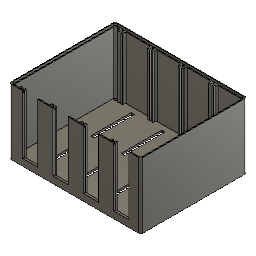
clusterbox-rock64-3d-v18 (Autodesk Fusion 360 design; units mm, degrees)
Autodesk Fusion 360 part; units mm, degrees
sketch "Sketch1" plane through (0, 0, 0) normal (0, 1, 0) x (1, 0, 0)
  line L0 (-65, -52.5) -> (65, -52.5)
  line L1 (65, -52.5) -> (65, 52.5)
  line L2 (65, 52.5) -> (-65, 52.5)
  line L3 (-65, 52.5) -> (-65, -52.5)
  line L4 (-65, -52.5) -> (65, 52.5) construction
  line L5 (65, -52.5) -> (-65, 52.5) construction
  dimension "d1" = 105
  dimension "d2" = 130
extrude "Extrude1" add sketch "Sketch1" along normal blind 65
sketch "Sketch2" plane through (0, 65, 0) normal (0, 1, 0) x (-1, 0, 0)
  line L0 (65, -52.5) -> (65, 52.5)
  line L1 (65, 52.5) -> (-65, 52.5)
  line L2 (-65, 52.5) -> (-65, -52.5)
  line L3 (-65, -52.5) -> (65, -52.5)
  line L4 (63, 50.5) -> (-63, 50.5)
  line L5 (-63, 50.5) -> (-63, -50.5)
  line L6 (-63, -50.5) -> (63, -50.5)
  line L7 (63, -50.5) -> (63, 50.5)
  line L8 (63, 50.5) -> (-63, -50.5) construction
  line L9 (-63, 50.5) -> (63, -50.5) construction
  dimension "d5" = 2
  dimension "d6" = 2
  measures "d5" distance of L0 L7
  measures "d6" distance of L1 L4
extrude "Extrude2" cut sketch "Sketch2" against normal blind 63 contours L4 L5 L6 L7
sketch "Sketch3" plane through (0, 2, 0) normal (0, 1, 0) x (-1, 0, 0)
  line L0 (63, -50.5) -> (63, 50.5)
  line L1 (63, 50.5) -> (-63, 50.5)
  line L2 (-63, 50.5) -> (-63, -50.5)
  line L3 (-63, -50.5) -> (63, -50.5)
  line L4 (58, -50.5) -> (53, -50.5)
  line L5 (53, -50.5) -> (53, -47.5)
  line L6 (53, -47.5) -> (58, -47.5)
  line L7 (58, -47.5) -> (58, -50.5)
  line L8 (63, 50.5) -> (63, -50.5)
  line L9 (65, -52.5) -> (65, 52.5) construction
  line L10 (-65, 52.5) -> (-65, -52.5) construction
  line L11 (65, 0) -> (-65, 0) construction
  line L12 (58, 50.5) -> (53, 50.5)
  line L13 (58, 47.5) -> (58, 50.5)
  line L14 (53, 47.5) -> (58, 47.5)
  line L15 (53, 50.5) -> (53, 47.5)
  dimension "d9" = 5
  dimension "d10" = 3
  dimension "d11" = 5
  measures "d11" distance of L7 L8
extrude "Extrude3" add sketch "Sketch3" along normal blind 63 contours L3 L4 L5 L6 L7 | L1 L12 L13 L14 L15
sketch "Sketch4" plane through (0, 2, 0) normal (0, 1, 0) x (-1, 0, 0)
  line L0 (58, 50.5) -> (58, 47.5)
  line L1 (58, 47.5) -> (53, 47.5)
  line L2 (53, 47.5) -> (53, 50.5)
  line L3 (53, 50.5) -> (-63, 50.5)
  line L4 (-63, 50.5) -> (-63, -50.5)
  line L5 (-63, -50.5) -> (53, -50.5)
  line L6 (53, -50.5) -> (53, -47.5)
  line L7 (53, -47.5) -> (58, -47.5)
  line L8 (58, -47.5) -> (58, -50.5)
  line L9 (58, -50.5) -> (63, -50.5)
  line L10 (63, -50.5) -> (63, 50.5)
  line L11 (63, 50.5) -> (58, 50.5)
  line L12 (56.375, -50.5) -> (54.625, -50.5)
  line L13 (54.625, -50.5) -> (54.625, 50.5)
  line L14 (54.625, 50.5) -> (56.375, 50.5)
  line L15 (56.375, 50.5) -> (56.375, -50.5)
  line L16 (0, 0) -> (54.625, 0) construction
  line L17 (58, -50.5) -> (58, -47.5) construction
  line L18 (55.5, -47.5) -> (55.5, -51.2811) construction
  dimension "d14" = 1.75
  dimension "d16" = 101
  measures "d14" distance of L13 L15
extrude "Extrude4" cut sketch "Sketch4" along normal blind 63 contours L1 L7 L13 L15 | L1 L13 L14 L15 | L7 L12 L13 L15
fillet "Fillet1" radius 1.5 4 edges at (-58, 33.5, 50.5) (-53, 33.5, 50.5) (-53, 33.5, -50.5) (-58, 33.5, -50.5)
pattern_linear "R-Pattern1" count 4 spacing 30 along (1, 0, 0) of "Extrude3", "Extrude4", "Fillet1"
fillet "Fillet2" radius 2 4 edges at (65, 32.5, -52.5) (65, 32.5, 52.5) (-65, 32.5, 52.5) (-65, 32.5, -52.5)
fillet "Fillet2" radius 2 4 edges at (63, 33.5, -50.5) (-63, 33.5, -50.5) (-63, 33.5, 50.5) (63, 33.5, 50.5)
sketch "Sketch5" plane through (0, 0, 0) normal (0, -1, 0) x (1, 0, 0)
  arc A0 (-65, -50.5) -> (-63, -52.5) centre (-63, -50.5) ccw
  line L0 (-63, -52.5) -> (63, -52.5)
  arc A1 (63, -52.5) -> (65, -50.5) centre (63, -50.5) ccw
  line L1 (65, -50.5) -> (65, 50.5)
  arc A2 (65, 50.5) -> (63, 52.5) centre (63, 50.5) ccw
  line L2 (63, 52.5) -> (-63, 52.5)
  arc A3 (-63, 52.5) -> (-65, 50.5) centre (-63, 50.5) ccw
  line L3 (-65, 50.5) -> (-65, -50.5)
  line L4 (-65, 48.5) -> (65, 48.5) construction
  line L5 (-65, 0) -> (65, 0) construction
  circle A4 centre (-61, 48.5) radius 1.1
  circle A5 centre (-61, -48.5) radius 1.1
  line L6 (0, 52.5) -> (0, 0) construction
  circle A6 centre (61, 48.5) radius 1.1
  circle A7 centre (61, -48.5) radius 1.1
  dimension "d29" = 2.2
  dimension "d36" = 4
  dimension "d37" = 4
  measures "d29" diameter of A4
extrude "Extrude5" cut sketch "Sketch5" against normal blind 2 contours A4 | A5 | A6 | A7
sketch "Sketch7" plane through (0, 2, 0) normal (0, 1, 0) x (-1, 0, 0)
  circle A0 centre (61, 48.5) radius 1.1
  circle A1 centre (61, -48.5) radius 1.1
  circle A2 centre (-61, 48.5) radius 1.1
  circle A3 centre (-61, -48.5) radius 1.1
  arc A4 (-61, 50.5) -> (-63, 48.5) centre (-61, 48.5) ccw
  line L0 (-63, 48.5) -> (-63, -48.5)
  arc A5 (-63, -48.5) -> (-61, -50.5) centre (-61, -48.5) ccw
  line L1 (-61, -50.5) -> (-38.5, -50.5)
  arc A6 (-38.5, -50.5) -> (-37, -49) centre (-38.5, -49) ccw
  line L2 (-37, -49) -> (-37, -47.5)
  line L3 (-37, -47.5) -> (-35.375, -47.5)
  line L4 (-35.375, -47.5) -> (-35.375, -50.5)
  line L5 (-35.375, -50.5) -> (-33.625, -50.5)
  line L6 (-33.625, -50.5) -> (-33.625, -47.5)
  line L7 (-33.625, -47.5) -> (-32, -47.5)
  line L8 (-32, -47.5) -> (-32, -49)
  arc A7 (-32, -49) -> (-30.5, -50.5) centre (-30.5, -49) ccw
  line L9 (-30.5, -50.5) -> (-8.5, -50.5)
  arc A8 (-8.5, -50.5) -> (-7, -49) centre (-8.5, -49) ccw
  line L10 (-7, -49) -> (-7, -47.5)
  line L11 (-7, -47.5) -> (-5.375, -47.5)
  line L12 (-5.375, -47.5) -> (-5.375, -50.5)
  line L13 (-5.375, -50.5) -> (-3.625, -50.5)
  line L14 (-3.625, -50.5) -> (-3.625, -47.5)
  line L15 (-3.625, -47.5) -> (-2, -47.5)
  line L16 (-2, -47.5) -> (-2, -49)
  arc A9 (-2, -49) -> (-0.5, -50.5) centre (-0.5, -49) ccw
  line L17 (-0.5, -50.5) -> (21.5, -50.5)
  arc A10 (21.5, -50.5) -> (23, -49) centre (21.5, -49) ccw
  line L18 (23, -49) -> (23, -47.5)
  line L19 (23, -47.5) -> (24.625, -47.5)
  line L20 (24.625, -47.5) -> (24.625, -50.5)
  line L21 (24.625, -50.5) -> (26.375, -50.5)
  line L22 (26.375, -50.5) -> (26.375, -47.5)
  line L23 (26.375, -47.5) -> (28, -47.5)
  line L24 (28, -47.5) -> (28, -49)
  arc A11 (28, -49) -> (29.5, -50.5) centre (29.5, -49) ccw
  line L25 (54.625, -47.5) -> (54.625, -50.5)
  line L26 (54.625, -50.5) -> (56.375, -50.5)
  line L27 (56.375, -50.5) -> (56.375, -47.5)
  line L28 (56.375, -47.5) -> (58, -47.5)
  line L29 (58, -47.5) -> (58, -49)
  arc A12 (58, -49) -> (59.5, -50.5) centre (59.5, -49) ccw
  line L30 (59.5, -50.5) -> (61, -50.5)
  arc A13 (61, -50.5) -> (63, -48.5) centre (61, -48.5) ccw
  line L31 (63, -48.5) -> (63, 48.5)
  arc A14 (63, 48.5) -> (61, 50.5) centre (61, 48.5) ccw
  line L32 (61, 50.5) -> (59.5, 50.5)
  arc A15 (59.5, 50.5) -> (58, 49) centre (59.5, 49) ccw
  line L33 (58, 49) -> (58, 47.5)
  line L34 (58, 47.5) -> (56.375, 47.5)
  line L35 (56.375, 47.5) -> (56.375, 50.5)
  line L36 (56.375, 50.5) -> (54.625, 50.5)
  line L37 (54.625, 50.5) -> (54.625, 47.5)
  arc A16 (29.5, 50.5) -> (28, 49) centre (29.5, 49) ccw
  line L38 (28, 49) -> (28, 47.5)
  line L39 (28, 47.5) -> (26.375, 47.5)
  line L40 (26.375, 47.5) -> (26.375, 50.5)
  line L41 (26.375, 50.5) -> (24.625, 50.5)
  line L42 (24.625, 50.5) -> (24.625, 47.5)
  line L43 (24.625, 47.5) -> (23, 47.5)
  line L44 (23, 47.5) -> (23, 49)
  arc A17 (23, 49) -> (21.5, 50.5) centre (21.5, 49) ccw
  line L45 (21.5, 50.5) -> (-0.5, 50.5)
  arc A18 (-0.5, 50.5) -> (-2, 49) centre (-0.5, 49) ccw
  line L46 (-2, 49) -> (-2, 47.5)
  line L47 (-2, 47.5) -> (-3.625, 47.5)
  line L48 (-3.625, 47.5) -> (-3.625, 50.5)
  line L49 (-3.625, 50.5) -> (-5.375, 50.5)
  line L50 (-5.375, 50.5) -> (-5.375, 47.5)
  line L51 (-5.375, 47.5) -> (-7, 47.5)
  line L52 (-7, 47.5) -> (-7, 49)
  arc A19 (-7, 49) -> (-8.5, 50.5) centre (-8.5, 49) ccw
  line L53 (-8.5, 50.5) -> (-30.5, 50.5)
  arc A20 (-30.5, 50.5) -> (-32, 49) centre (-30.5, 49) ccw
  line L54 (-32, 49) -> (-32, 47.5)
  line L55 (-32, 47.5) -> (-33.625, 47.5)
  line L56 (-33.625, 47.5) -> (-33.625, 50.5)
  line L57 (-33.625, 50.5) -> (-35.375, 50.5)
  line L58 (-35.375, 50.5) -> (-35.375, 47.5)
  line L59 (-35.375, 47.5) -> (-37, 47.5)
  line L60 (-37, 47.5) -> (-37, 49)
  arc A21 (-37, 49) -> (-38.5, 50.5) centre (-38.5, 49) ccw
  line L61 (-38.5, 50.5) -> (-61, 50.5)
  line L62 (63, 0) -> (-63, 0) construction
  line L63 (51.5, -50.5) -> (29.5, -50.5) construction
  line L64 (40.5, -50.5) -> (40.5, 0) construction
  line L65 (42.1, -5.25) -> (38.9, -5.25)
  line L66 (38.9, -5.25) -> (38.9, -45.25)
  line L67 (38.9, -45.25) -> (42.1, -45.25)
  line L68 (42.1, -45.25) -> (42.1, -5.25)
  line L69 (42.1, -5.25) -> (38.9, -45.25) construction
  line L70 (38.9, -5.25) -> (42.1, -45.25) construction
  line L71 (42.1, 45.25) -> (42.1, 5.25)
  line L72 (38.9, 45.25) -> (42.1, 45.25)
  line L73 (38.9, 5.25) -> (38.9, 45.25)
  line L74 (42.1, 5.25) -> (38.9, 5.25)
  dimension "d51" = 3.2
  dimension "d52" = 40
  measures "d52" distance of origin
extrude "Extrude6" cut sketch "Sketch7" against normal through all contours L65 L66 L67 L68 | L71 L72 L73 L74
pattern_linear "R-Pattern2" count 4 spacing 30 along (1, 0, 0) of "Extrude6"
sketch "Sketch6" plane through (0, 65, 0) normal (0, 1, 0) x (-1, 0, 0)
  arc A0 (63, -52.5) -> (65, -50.5) centre (63, -50.5) ccw
  line L0 (65, -50.5) -> (65, 50.5)
  arc A1 (65, 50.5) -> (63, 52.5) centre (63, 50.5) ccw
  line L1 (63, 52.5) -> (-63, 52.5)
  arc A2 (-63, 52.5) -> (-65, 50.5) centre (-63, 50.5) ccw
  line L2 (-65, 50.5) -> (-65, -50.5)
  arc A3 (-65, -50.5) -> (-63, -52.5) centre (-63, -50.5) ccw
  line L3 (-63, -52.5) -> (63, -52.5)
  line L4 (-33.625, -47.5) -> (-33.625, -50.5)
  line L5 (-33.625, -50.5) -> (-35.375, -50.5)
  line L6 (-35.375, -50.5) -> (-35.375, -47.5)
  line L7 (-35.375, -47.5) -> (-37, -47.5)
  line L8 (-37, -47.5) -> (-37, -49)
  arc A4 (-38.5, -50.5) -> (-37, -49) centre (-38.5, -49) ccw
  line L9 (-38.5, -50.5) -> (-61, -50.5)
  arc A5 (-63, -48.5) -> (-61, -50.5) centre (-61, -48.5) ccw
  line L10 (-63, -48.5) -> (-63, 48.5)
  arc A6 (-61, 50.5) -> (-63, 48.5) centre (-61, 48.5) ccw
  line L11 (-61, 50.5) -> (-38.5, 50.5)
  arc A7 (-37, 49) -> (-38.5, 50.5) centre (-38.5, 49) ccw
  line L12 (-37, 49) -> (-37, 47.5)
  line L13 (-37, 47.5) -> (-35.375, 47.5)
  line L14 (-35.375, 47.5) -> (-35.375, 50.5)
  line L15 (-35.375, 50.5) -> (-33.625, 50.5)
  line L16 (-33.625, 50.5) -> (-33.625, 47.5)
  line L17 (-33.625, 47.5) -> (-32, 47.5)
  line L18 (-32, 47.5) -> (-32, 49)
  arc A8 (-30.5, 50.5) -> (-32, 49) centre (-30.5, 49) ccw
  line L19 (-30.5, 50.5) -> (-8.5, 50.5)
  arc A9 (-7, 49) -> (-8.5, 50.5) centre (-8.5, 49) ccw
  line L20 (-7, 49) -> (-7, 47.5)
  line L21 (-7, 47.5) -> (-5.375, 47.5)
  line L22 (-5.375, 47.5) -> (-5.375, 50.5)
  line L23 (-5.375, 50.5) -> (-3.625, 50.5)
  line L24 (-3.625, 50.5) -> (-3.625, 47.5)
  line L25 (-3.625, 47.5) -> (-2, 47.5)
  line L26 (-2, 47.5) -> (-2, 49)
  arc A10 (-0.5, 50.5) -> (-2, 49) centre (-0.5, 49) ccw
  line L27 (-0.5, 50.5) -> (21.5, 50.5)
  arc A11 (23, 49) -> (21.5, 50.5) centre (21.5, 49) ccw
  line L28 (23, 49) -> (23, 47.5)
  line L29 (23, 47.5) -> (24.625, 47.5)
  line L30 (24.625, 47.5) -> (24.625, 50.5)
  line L31 (24.625, 50.5) -> (26.375, 50.5)
  line L32 (26.375, 50.5) -> (26.375, 47.5)
  line L33 (26.375, 47.5) -> (28, 47.5)
  line L34 (28, 47.5) -> (28, 49)
  arc A12 (29.5, 50.5) -> (28, 49) centre (29.5, 49) ccw
  line L35 (29.5, 50.5) -> (51.5, 50.5)
  arc A13 (53, 49) -> (51.5, 50.5) centre (51.5, 49) ccw
  line L36 (53, 49) -> (53, 47.5)
  line L37 (53, 47.5) -> (54.625, 47.5)
  line L38 (54.625, 47.5) -> (54.625, 50.5)
  line L39 (54.625, 50.5) -> (56.375, 50.5)
  line L40 (56.375, 50.5) -> (56.375, 47.5)
  line L41 (56.375, 47.5) -> (58, 47.5)
  line L42 (58, 47.5) -> (58, 49)
  arc A14 (59.5, 50.5) -> (58, 49) centre (59.5, 49) ccw
  line L43 (59.5, 50.5) -> (61, 50.5)
  arc A15 (63, 48.5) -> (61, 50.5) centre (61, 48.5) ccw
  line L44 (63, 48.5) -> (63, -48.5)
  arc A16 (61, -50.5) -> (63, -48.5) centre (61, -48.5) ccw
  line L45 (61, -50.5) -> (59.5, -50.5)
  arc A17 (58, -49) -> (59.5, -50.5) centre (59.5, -49) ccw
  line L46 (58, -49) -> (58, -47.5)
  line L47 (58, -47.5) -> (56.375, -47.5)
  line L48 (56.375, -47.5) -> (56.375, -50.5)
  line L49 (56.375, -50.5) -> (54.625, -50.5)
  line L50 (54.625, -50.5) -> (54.625, -47.5)
  line L51 (54.625, -47.5) -> (53, -47.5)
  line L52 (53, -47.5) -> (53, -49)
  arc A18 (51.5, -50.5) -> (53, -49) centre (51.5, -49) ccw
  line L53 (51.5, -50.5) -> (29.5, -50.5)
  arc A19 (28, -49) -> (29.5, -50.5) centre (29.5, -49) ccw
  line L54 (28, -49) -> (28, -47.5)
  line L55 (28, -47.5) -> (26.375, -47.5)
  line L56 (26.375, -47.5) -> (26.375, -50.5)
  line L57 (26.375, -50.5) -> (24.625, -50.5)
  line L58 (24.625, -50.5) -> (24.625, -47.5)
  line L59 (24.625, -47.5) -> (23, -47.5)
  line L60 (23, -47.5) -> (23, -49)
  arc A20 (21.5, -50.5) -> (23, -49) centre (21.5, -49) ccw
  line L61 (21.5, -50.5) -> (-0.5, -50.5)
  arc A21 (-2, -49) -> (-0.5, -50.5) centre (-0.5, -49) ccw
  line L62 (-2, -49) -> (-2, -47.5)
  line L63 (-2, -47.5) -> (-3.625, -47.5)
  line L64 (-3.625, -47.5) -> (-3.625, -50.5)
  line L65 (-3.625, -50.5) -> (-5.375, -50.5)
  line L66 (-5.375, -50.5) -> (-5.375, -47.5)
  line L67 (-5.375, -47.5) -> (-7, -47.5)
  line L68 (-7, -47.5) -> (-7, -49)
  arc A22 (-8.5, -50.5) -> (-7, -49) centre (-8.5, -49) ccw
  line L69 (-8.5, -50.5) -> (-30.5, -50.5)
  arc A23 (-32, -49) -> (-30.5, -50.5) centre (-30.5, -49) ccw
  line L70 (-32, -49) -> (-32, -47.5)
  line L71 (-32, -47.5) -> (-33.625, -47.5)
  line L72 (-62, -51.5) -> (62, -51.5)
  line L73 (64, -49.5) -> (64, 49.5)
  line L74 (62, 51.5) -> (-62, 51.5)
  line L75 (-64, 49.5) -> (-64, -49.5)
  line L76 (-64, -51.5) -> (64, 51.5) construction
  line L77 (64, -51.5) -> (-64, 51.5) construction
  arc A24 (62, -51.5) -> (64, -49.5) centre (62, -49.5) ccw
  arc A25 (64, 49.5) -> (62, 51.5) centre (62, 49.5) ccw
  arc A26 (-64, -49.5) -> (-62, -51.5) centre (-62, -49.5) ccw
  arc A27 (-62, 51.5) -> (-64, 49.5) centre (-62, 49.5) ccw
  dimension "d34" = 1
  dimension "d35" = 1
  dimension "d45" = 2
  dimension "d46" = 2
  dimension "d47" = 2
  dimension "d48" = 2
  measures "d34" distance of L3 L72
  measures "d35" distance of L2 L75
  measures "d45" radius of A24
  measures "d46" radius of A25
  measures "d47" radius of A26
  measures "d48" radius of A27
extrude "Extrude7" cut sketch "Sketch6" against normal blind 2 contours L72 L73 L74 L75 A24 A25 A26 A27
sketch "Sketch9" plane through (0, 0, 50.5) normal (0, 0, -1) x (-1, 0, 0)
  line L0 (51.5, 63) -> (29.5, 63)
  line L1 (29.5, 63) -> (29.5, 2)
  line L2 (29.5, 2) -> (51.5, 2)
  line L3 (51.5, 2) -> (51.5, 63)
  line L4 (39.6847, 85) -> (48.5653, 85)
  line L5 (51.625, 81.9403) -> (51.625, 7)
  line L6 (51.625, 7) -> (36.625, 7)
  line L7 (36.625, 7) -> (36.625, 81.9403)
  line L8 (54.625, 2) -> (54.625, 63)
  arc A0 (39.6847, 85) -> (36.625, 81.9403) centre (39.6847, 81.9403) ccw
  arc A1 (51.625, 81.9403) -> (48.5653, 85) centre (48.5653, 81.9403) ccw
  line L9 (-62, 65) -> (62, 65)
  dimension "d53" = 15
  dimension "d55" = 3
  dimension "d56" = 5
  dimension "d65" = 20
  measures "d55" distance of L5 L8
  measures "d56" distance of L2 L6
  measures "d65" distance of L4 L9
extrude "Extrude8" cut sketch "Sketch9" against normal through all contours L0 L3 L6 L7 | L0 L3 L5 L6 L7 L9 | L4 L5 L7 A0 A1 L9
pattern_linear "R-Pattern3" count 4 spacing 30 along (1, 0, 0) of "Extrude8"
equation "d2 = ( 32.5 * 4 ) * 1 mm"
